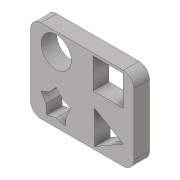
# Autodesk Inventor part: PassengerBaseNT
Saved by Autodesk Inventor 2016 (Build 200138000, 138)
## iProperties
Created: 2016-01-13
Part Number: PassengerBaseNT
Material: Generic
Document SubType Name: Modeling
Designer: 301278
Density: 1 g/cm^3
Appearance: Default
Author: 301278
Autodesk Inventor part; units mm, degrees
ref_plane "YZ Plane" through (0, 0, 0) normal (1, 0, 0) x (0, 1, 0)
ref_plane "XZ Plane" through (0, 0, 0) normal (0, 1, 0) x (-1, 0, 0)
ref_plane "XY Plane" through (0, 0, 0) normal (0, 0, 1) x (1, 0, 0)
sketch "Sketch1" plane through (0, 0, 0) normal (0, 0, 1) x (1, 0, 0)
  line L0 (0, 0) -> (50.165, 0)
  line L1 (50.165, 0) -> (50.165, 40.386)
  line L2 (50.165, 40.386) -> (0, 40.386)
  line L3 (0, 40.386) -> (0, 0)
  dimension "d0" = 50.165
  dimension "d1" = 40.386
  constraints: 8 end point, 2 parallel, 1 horizontal, 1 perpendicular
  measures "d0" distance of L2.end L1.end
  measures "d1" distance of L1.end L0.end
extrude "Extrusion1" add sketch "Sketch1" along normal blind 7.62
sketch "Sketch2" plane through (0, 0, 7.62) normal (0, 0, 1) x (1, 0, 0)
  circle A0 centre (12.446, 31.75) radius 7.366
  line L0 (0, 40.386) -> (0, 0) projected
  line L1 (50.165, 40.386) -> (0, 40.386) projected
  line L2 (30.353, 39.116) -> (45.085, 39.116)
  line L3 (45.085, 39.116) -> (45.085, 24.384)
  line L4 (45.085, 24.384) -> (30.353, 24.384)
  line L5 (30.353, 24.384) -> (30.353, 39.116)
  line L6 (50.165, 0) -> (50.165, 40.386) projected
  line L7 (31.0509, 1.27) -> (31.0509, 17.4752)
  line L8 (31.0509, 17.4752) -> (45.085, 9.3726)
  line L9 (45.085, 9.3726) -> (31.0509, 1.27)
  line L10 (0, 0) -> (50.165, 0) projected
  circle A1 centre (12.3952, 9.2202) radius 7.6835 construction
  line L11 (12.3952, 16.9037) -> (19.7026, 11.5945) construction
  line L12 (19.7026, 11.5945) -> (16.9114, 3.0041) construction
  line L13 (16.9114, 3.0041) -> (7.879, 3.0041) construction
  line L14 (7.879, 3.0041) -> (5.0878, 11.5945) construction
  line L15 (5.0878, 11.5945) -> (12.3952, 16.9037) construction
  circle A2 centre (12.3952, 9.2202) radius 5.2324 construction
  line L16 (12.3952, 16.9037) -> (9.3197, 13.4533)
  line L17 (9.3197, 13.4533) -> (5.0878, 11.5945)
  line L18 (5.0878, 11.5945) -> (7.4189, 7.6033)
  line L19 (7.4189, 7.6033) -> (7.879, 3.0041)
  line L20 (7.879, 3.0041) -> (12.3952, 3.9878)
  line L21 (16.9114, 3.0041) -> (12.3952, 3.9878)
  line L22 (16.9114, 3.0041) -> (17.3715, 7.6033)
  line L23 (17.3715, 7.6033) -> (19.7026, 11.5945)
  line L24 (12.3952, 16.9037) -> (15.4707, 13.4533)
  line L25 (19.7026, 11.5945) -> (15.4707, 13.4533)
  point P0 (35.7289, 9.3726)
  dimension "d4" = 14.732
  dimension "d5" = 12.446
  dimension "d6" = 8.636
  dimension "d7" = 14.732
  dimension "d8" = 5.08
  dimension "d9" = 1.27
  dimension "d10" = 14.732
  dimension "d11" = 16.2052
  dimension "d12" = 1.27
  dimension "d13" = 5.08
  dimension "d14" = 15.367
  dimension "d15" = 12.3952
  dimension "d16" = 9.2202
  dimension "d17" = 10.4648
  constraints: 44 end point, 7 point on circle, 5 equal length, 3 centre point, 2 coincident, 2 parallel, 1 horizontal, 1 perpendicular, 1 point on line, 1 vertical, 18 other
  measures "d4" diameter of A0
  measures "d5" distance from line of A0.centre L0
  measures "d6" distance from line of A0.centre L1
  measures "d7" distance of L2.end L2.start
  measures "d8" distance between parallel lines of L6 L3
  measures "d9" distance between parallel lines of L1 L2
  measures "d10" distance between parallel lines of L2 L4
  measures "d11" distance of L7.start L7.end
  measures "d12" distance from line of L10 L7.start
  measures "d13" distance from line of L6 L8.end
  measures "d14" diameter of A1
  measures "d15" distance from line of L0 A1.centre
  measures "d16" distance from line of L10 A1.centre
  measures "d17" diameter of A2
extrude "Extrusion2" cut sketch "Sketch2" against normal blind 25.4 contours A0 | L2 L3 L4 L5 | L7 L8 L9 | L24 L25 L23 L22 L21 L20 L19 L18 L17 L16
fillet "Fillet1" radius 5.08 1 edges at (50.165, 40.386, 3.81)
fillet "Fillet2" radius 5.08 1 edges at (0, 40.386, 3.81)
fillet "Fillet3" radius 5.08 1 edges at (50.165, 0, 3.81)
fillet "Fillet4" radius 5.08 1 edges at (0, 0, 3.81)
shell "Shell1" thickness 0.254 removed faces 1 at (40.407, 17.0773, 0)
body "Solid1"
